Autodesk Fusion 360 part; units mm, degrees
note: some values were not read from the file. Set by a fixed rule: which face or edge a step refers to.
(part 2 of 5)
sketch "Sketch5" plane through (10, 0, 0) normal (1, 0, 0) x (0, 1, 0)
  arc A0 (-151.958, 246.6024) -> (-148.4708, 246.6024) centre (-150.2144, 250.2024) ccw
  line L0 (-151.958, 246.6024) -> (-300.2144, 246.6024)
  line L1 (-300.2144, 246.6024) -> (-300.2144, 240.2024)
  line L2 (-300.2144, 240.2024) -> (249.7856, 240.2024)
  line L3 (249.7856, 240.2024) -> (249.7856, 246.6024)
  line L4 (249.7856, 246.6024) -> (-148.4708, 246.6024)
  line L5 (59.7856, 246.6024) -> (59.7856, 240.2024)
  line L6 (226.7856, 240.2024) -> (226.7856, 243.4024)
  line L7 (235.7856, 240.2024) -> (235.7856, 243.4024)
  line L8 (219.7856, 246.6024) -> (219.7856, 240.2024)
  line L9 (-20.2144, 246.6024) -> (-20.2144, 240.2024)
  line L10 (69.7856, 246.6024) -> (69.7856, 240.2024)
  line L11 (209.7856, 246.6024) -> (209.7856, 240.2024)
  line L12 (-0.2144, 246.6024) -> (-0.2144, 240.2024)
  line L13 (-10.2144, 246.6024) -> (-10.2144, 240.2024)
  line L14 (239.7856, 246.6024) -> (239.7856, 240.2024)
  line L15 (39.7856, 246.6024) -> (39.7856, 240.2024)
  line L16 (232.7856, 240.2024) -> (232.7856, 243.4024)
  line L17 (149.7856, 246.6024) -> (149.7856, 240.2024)
  line L18 (-40.2144, 246.6024) -> (-40.2144, 240.2024)
  line L19 (-50.2144, 246.6024) -> (-50.2144, 240.2024)
  line L20 (29.7856, 246.6024) -> (29.7856, 240.2024)
  line L21 (199.7856, 246.6024) -> (199.7856, 240.2024)
  line L22 (129.7856, 246.6024) -> (129.7856, 240.2024)
  line L23 (224.7856, 240.2024) -> (224.7856, 243.4024)
  line L24 (237.7856, 240.2024) -> (237.7856, 243.4024)
  line L25 (49.7856, 246.6024) -> (49.7856, 240.2024)
  line L26 (218.7856, 240.2024) -> (218.7856, 243.4024)
  line L27 (19.7856, 246.6024) -> (19.7856, 240.2024)
  line L28 (249.7856, 240.2024) -> (249.7856, 246.6024)
  line L29 (159.7856, 246.6024) -> (159.7856, 240.2024)
  line L30 (229.7856, 246.6024) -> (229.7856, 240.2024)
  line L31 (99.7856, 246.6024) -> (99.7856, 240.2024)
  line L32 (249.7856, 246.6024) -> (-120.2144, 246.6024)
  line L33 (169.7856, 246.6024) -> (169.7856, 240.2024)
  line L34 (139.7856, 246.6024) -> (139.7856, 240.2024)
  line L35 (-30.2144, 246.6024) -> (-30.2144, 240.2024)
  line L36 (119.7856, 246.6024) -> (119.7856, 240.2024)
  line L37 (9.7856, 246.6024) -> (9.7856, 240.2024)
  line L38 (-120.2144, 246.6024) -> (-120.2144, 240.2024)
  line L39 (241.7856, 240.2024) -> (241.7856, 243.4024)
  line L40 (231.7856, 240.2024) -> (231.7856, 243.4024)
  line L41 (179.7856, 246.6024) -> (179.7856, 240.2024)
  line L42 (-120.2144, 240.2024) -> (249.7856, 240.2024)
  line L43 (109.7856, 246.6024) -> (109.7856, 240.2024)
  line L44 (189.7856, 246.6024) -> (189.7856, 240.2024)
  line L45 (89.7856, 246.6024) -> (89.7856, 240.2024)
  line L46 (79.7856, 246.6024) -> (79.7856, 240.2024)
  line L47 (205.7856, 240.2024) -> (205.7856, 243.4024)
  line L48 (193.7856, 240.2024) -> (193.7856, 243.4024)
  line L49 (199.7856, 240.2024) -> (199.7856, 243.4024)
  line L50 (238.7856, 240.2024) -> (238.7856, 243.4024)
  line L51 (247.7856, 240.2024) -> (247.7856, 243.4024)
  line L52 (204.7856, 240.2024) -> (204.7856, 243.4024)
  line L53 (223.7856, 240.2024) -> (223.7856, 243.4024)
  line L54 (-90.2144, 246.6024) -> (-90.2144, 240.2024)
  line L55 (215.7856, 240.2024) -> (215.7856, 243.4024)
  line L56 (-70.2144, 246.6024) -> (-70.2144, 240.2024)
  line L57 (246.7856, 240.2024) -> (246.7856, 243.4024)
  line L58 (201.7856, 240.2024) -> (201.7856, 243.4024)
  line L59 (200.7856, 240.2024) -> (200.7856, 243.4024)
  line L60 (245.7856, 240.2024) -> (245.7856, 243.4024)
  line L61 (227.7856, 240.2024) -> (227.7856, 243.4024)
  line L62 (244.7856, 240.2024) -> (244.7856, 243.4024)
  line L63 (140.7856, 240.2024) -> (140.7856, 243.4024)
  line L64 (203.7856, 240.2024) -> (203.7856, 243.4024)
  line L65 (197.7856, 240.2024) -> (197.7856, 243.4024)
  line L66 (211.7856, 240.2024) -> (211.7856, 243.4024)
  line L67 (212.7856, 240.2024) -> (212.7856, 243.4024)
  line L68 (219.7856, 240.2024) -> (219.7856, 243.4024)
  line L69 (198.7856, 240.2024) -> (198.7856, 243.4024)
  line L70 (234.7856, 240.2024) -> (234.7856, 243.4024)
  line L71 (230.7856, 240.2024) -> (230.7856, 243.4024)
  line L72 (202.7856, 240.2024) -> (202.7856, 243.4024)
  line L73 (248.7856, 240.2024) -> (248.7856, 243.4024)
  line L74 (192.7856, 240.2024) -> (192.7856, 243.4024)
  line L75 (249.7856, 240.2024) -> (249.7856, 243.4024)
  line L76 (242.7856, 240.2024) -> (242.7856, 243.4024)
  line L77 (214.7856, 240.2024) -> (214.7856, 243.4024)
  line L78 (243.7856, 240.2024) -> (243.7856, 243.4024)
  line L79 (194.7856, 240.2024) -> (194.7856, 243.4024)
  line L80 (216.7856, 240.2024) -> (216.7856, 243.4024)
  line L81 (-100.2144, 246.6024) -> (-100.2144, 240.2024)
  line L82 (196.7856, 240.2024) -> (196.7856, 243.4024)
  line L83 (208.7856, 240.2024) -> (208.7856, 243.4024)
  line L84 (228.7856, 240.2024) -> (228.7856, 243.4024)
  line L85 (181.7856, 240.2024) -> (181.7856, 243.4024)
  line L86 (171.7856, 240.2024) -> (171.7856, 243.4024)
  line L87 (160.7856, 240.2024) -> (160.7856, 243.4024)
  line L88 (169.7856, 240.2024) -> (169.7856, 243.4024)
  line L89 (151.7856, 240.2024) -> (151.7856, 243.4024)
  line L90 (220.7856, 240.2024) -> (220.7856, 243.4024)
  line L91 (210.7856, 240.2024) -> (210.7856, 243.4024)
  line L92 (185.7856, 240.2024) -> (185.7856, 243.4024)
  line L93 (240.7856, 240.2024) -> (240.7856, 243.4024)
  line L94 (217.7856, 240.2024) -> (217.7856, 243.4024)
  line L95 (233.7856, 240.2024) -> (233.7856, 243.4024)
  line L96 (225.7856, 240.2024) -> (225.7856, 243.4024)
  line L97 (207.7856, 240.2024) -> (207.7856, 243.4024)
  line L98 (158.7856, 240.2024) -> (158.7856, 243.4024)
  line L99 (222.7856, 240.2024) -> (222.7856, 243.4024)
  line L100 (209.7856, 240.2024) -> (209.7856, 243.4024)
  line L101 (-60.2144, 246.6024) -> (-60.2144, 240.2024)
  line L102 (221.7856, 240.2024) -> (221.7856, 243.4024)
  line L103 (-110.2144, 246.6024) -> (-110.2144, 240.2024)
  line L104 (239.7856, 240.2024) -> (239.7856, 243.4024)
  line L105 (-80.2144, 246.6024) -> (-80.2144, 240.2024)
  line L106 (236.7856, 240.2024) -> (236.7856, 243.4024)
  line L107 (229.7856, 240.2024) -> (229.7856, 243.4024)
  line L108 (213.7856, 240.2024) -> (213.7856, 243.4024)
  line L109 (206.7856, 240.2024) -> (206.7856, 243.4024)
  line L110 (195.7856, 240.2024) -> (195.7856, 243.4024)
  line L111 (131.7856, 240.2024) -> (131.7856, 243.4024)
  line L112 (129.7856, 240.2024) -> (129.7856, 243.4024)
  line L113 (177.7856, 240.2024) -> (177.7856, 243.4024)
  line L114 (174.7856, 240.2024) -> (174.7856, 243.4024)
  line L115 (183.7856, 240.2024) -> (183.7856, 243.4024)
  line L116 (179.7856, 240.2024) -> (179.7856, 243.4024)
  line L117 (180.7856, 240.2024) -> (180.7856, 243.4024)
  line L118 (155.7856, 240.2024) -> (155.7856, 243.4024)
  line L119 (191.7856, 240.2024) -> (191.7856, 243.4024)
  line L120 (152.7856, 240.2024) -> (152.7856, 243.4024)
  line L121 (130.7856, 240.2024) -> (130.7856, 243.4024)
  line L122 (190.7856, 240.2024) -> (190.7856, 243.4024)
  line L123 (170.7856, 240.2024) -> (170.7856, 243.4024)
  line L124 (91.7856, 240.2024) -> (91.7856, 243.4024)
  line L125 (122.7856, 240.2024) -> (122.7856, 243.4024)
  line L126 (143.7856, 240.2024) -> (143.7856, 243.4024)
  line L127 (132.7856, 240.2024) -> (132.7856, 243.4024)
  line L128 (184.7856, 240.2024) -> (184.7856, 243.4024)
  line L129 (161.7856, 240.2024) -> (161.7856, 243.4024)
  line L130 (96.7856, 240.2024) -> (96.7856, 243.4024)
  line L131 (84.7856, 240.2024) -> (84.7856, 243.4024)
  line L132 (82.7856, 240.2024) -> (82.7856, 243.4024)
  line L133 (172.7856, 240.2024) -> (172.7856, 243.4024)
  line L134 (92.7856, 240.2024) -> (92.7856, 243.4024)
  line L135 (144.7856, 240.2024) -> (144.7856, 243.4024)
  line L136 (147.7856, 240.2024) -> (147.7856, 243.4024)
  line L137 (81.7856, 240.2024) -> (81.7856, 243.4024)
  line L138 (138.7856, 240.2024) -> (138.7856, 243.4024)
  line L139 (86.7856, 240.2024) -> (86.7856, 243.4024)
  line L140 (149.7856, 240.2024) -> (149.7856, 243.4024)
  line L141 (175.7856, 240.2024) -> (175.7856, 243.4024)
  line L142 (176.7856, 240.2024) -> (176.7856, 243.4024)
  line L143 (182.7856, 240.2024) -> (182.7856, 243.4024)
  line L144 (137.7856, 240.2024) -> (137.7856, 243.4024)
  line L145 (156.7856, 240.2024) -> (156.7856, 243.4024)
  line L146 (128.7856, 240.2024) -> (128.7856, 243.4024)
  line L147 (135.7856, 240.2024) -> (135.7856, 243.4024)
  line L148 (136.7856, 240.2024) -> (136.7856, 243.4024)
  line L149 (167.7856, 240.2024) -> (167.7856, 243.4024)
  line L150 (142.7856, 240.2024) -> (142.7856, 243.4024)
  line L151 (189.7856, 240.2024) -> (189.7856, 243.4024)
  line L152 (133.7856, 240.2024) -> (133.7856, 243.4024)
  line L153 (145.7856, 240.2024) -> (145.7856, 243.4024)
  line L154 (157.7856, 240.2024) -> (157.7856, 243.4024)
  line L155 (173.7856, 240.2024) -> (173.7856, 243.4024)
  line L156 (165.7856, 240.2024) -> (165.7856, 243.4024)
  line L157 (153.7856, 240.2024) -> (153.7856, 243.4024)
  line L158 (159.7856, 240.2024) -> (159.7856, 243.4024)
  line L159 (141.7856, 240.2024) -> (141.7856, 243.4024)
  line L160 (134.7856, 240.2024) -> (134.7856, 243.4024)
  line L161 (166.7856, 240.2024) -> (166.7856, 243.4024)
  line L162 (178.7856, 240.2024) -> (178.7856, 243.4024)
  line L163 (146.7856, 240.2024) -> (146.7856, 243.4024)
  line L164 (186.7856, 240.2024) -> (186.7856, 243.4024)
  line L165 (188.7856, 240.2024) -> (188.7856, 243.4024)
  line L166 (148.7856, 240.2024) -> (148.7856, 243.4024)
  line L167 (154.7856, 240.2024) -> (154.7856, 243.4024)
  line L168 (162.7856, 240.2024) -> (162.7856, 243.4024)
  line L169 (168.7856, 240.2024) -> (168.7856, 243.4024)
  line L170 (164.7856, 240.2024) -> (164.7856, 243.4024)
  line L171 (187.7856, 240.2024) -> (187.7856, 243.4024)
  line L172 (139.7856, 240.2024) -> (139.7856, 243.4024)
  line L173 (150.7856, 240.2024) -> (150.7856, 243.4024)
  line L174 (163.7856, 240.2024) -> (163.7856, 243.4024)
  line L175 (73.7856, 240.2024) -> (73.7856, 243.4024)
  line L176 (71.7856, 240.2024) -> (71.7856, 243.4024)
  line L177 (77.7856, 240.2024) -> (77.7856, 243.4024)
  line L178 (70.7856, 240.2024) -> (70.7856, 243.4024)
  line L179 (88.7856, 240.2024) -> (88.7856, 243.4024)
  line L180 (85.7856, 240.2024) -> (85.7856, 243.4024)
  line L181 (67.7856, 240.2024) -> (67.7856, 243.4024)
  line L182 (99.7856, 240.2024) -> (99.7856, 243.4024)
  line L183 (98.7856, 240.2024) -> (98.7856, 243.4024)
  line L184 (68.7856, 240.2024) -> (68.7856, 243.4024)
  line L185 (87.7856, 240.2024) -> (87.7856, 243.4024)
  line L186 (120.7856, 240.2024) -> (120.7856, 243.4024)
  line L187 (112.7856, 240.2024) -> (112.7856, 243.4024)
  line L188 (101.7856, 240.2024) -> (101.7856, 243.4024)
  line L189 (104.7856, 240.2024) -> (104.7856, 243.4024)
  line L190 (64.7856, 240.2024) -> (64.7856, 243.4024)
  line L191 (72.7856, 240.2024) -> (72.7856, 243.4024)
  line L192 (78.7856, 240.2024) -> (78.7856, 243.4024)
  line L193 (127.7856, 240.2024) -> (127.7856, 243.4024)
  line L194 (49.7856, 240.2024) -> (49.7856, 243.4024)
  line L195 (36.7856, 240.2024) -> (36.7856, 243.4024)
  line L196 (62.7856, 240.2024) -> (62.7856, 243.4024)
  line L197 (119.7856, 240.2024) -> (119.7856, 243.4024)
  line L198 (39.7856, 240.2024) -> (39.7856, 243.4024)
  line L199 (65.7856, 240.2024) -> (65.7856, 243.4024)
  line L200 (56.7856, 240.2024) -> (56.7856, 243.4024)
  line L201 (28.7856, 240.2024) -> (28.7856, 243.4024)
  line L202 (51.7856, 240.2024) -> (51.7856, 243.4024)
  line L203 (54.7856, 240.2024) -> (54.7856, 243.4024)
  line L204 (126.7856, 240.2024) -> (126.7856, 243.4024)
  line L205 (116.7856, 240.2024) -> (116.7856, 243.4024)
  line L206 (110.7856, 240.2024) -> (110.7856, 243.4024)
  line L207 (102.7856, 240.2024) -> (102.7856, 243.4024)
  line L208 (95.7856, 240.2024) -> (95.7856, 243.4024)
  line L209 (79.7856, 240.2024) -> (79.7856, 243.4024)
  line L210 (117.7856, 240.2024) -> (117.7856, 243.4024)
  line L211 (69.7856, 240.2024) -> (69.7856, 243.4024)
  line L212 (124.7856, 240.2024) -> (124.7856, 243.4024)
  line L213 (80.7856, 240.2024) -> (80.7856, 243.4024)
  line L214 (123.7856, 240.2024) -> (123.7856, 243.4024)
  line L215 (107.7856, 240.2024) -> (107.7856, 243.4024)
  line L216 (66.7856, 240.2024) -> (66.7856, 243.4024)
  line L217 (113.7856, 240.2024) -> (113.7856, 243.4024)
  line L218 (76.7856, 240.2024) -> (76.7856, 243.4024)
  line L219 (89.7856, 240.2024) -> (89.7856, 243.4024)
  line L220 (105.7856, 240.2024) -> (105.7856, 243.4024)
  line L221 (121.7856, 240.2024) -> (121.7856, 243.4024)
  line L222 (106.7856, 240.2024) -> (106.7856, 243.4024)
  line L223 (118.7856, 240.2024) -> (118.7856, 243.4024)
  line L224 (109.7856, 240.2024) -> (109.7856, 243.4024)
  line L225 (115.7856, 240.2024) -> (115.7856, 243.4024)
  line L226 (114.7856, 240.2024) -> (114.7856, 243.4024)
  line L227 (94.7856, 240.2024) -> (94.7856, 243.4024)
  line L228 (74.7856, 240.2024) -> (74.7856, 243.4024)
  line L229 (93.7856, 240.2024) -> (93.7856, 243.4024)
  line L230 (111.7856, 240.2024) -> (111.7856, 243.4024)
  line L231 (75.7856, 240.2024) -> (75.7856, 243.4024)
  line L232 (103.7856, 240.2024) -> (103.7856, 243.4024)
  line L233 (83.7856, 240.2024) -> (83.7856, 243.4024)
  line L234 (125.7856, 240.2024) -> (125.7856, 243.4024)
  line L235 (97.7856, 240.2024) -> (97.7856, 243.4024)
  line L236 (100.7856, 240.2024) -> (100.7856, 243.4024)
  line L237 (90.7856, 240.2024) -> (90.7856, 243.4024)
  line L238 (108.7856, 240.2024) -> (108.7856, 243.4024)
  line L239 (24.7856, 240.2024) -> (24.7856, 243.4024)
  line L240 (19.7856, 240.2024) -> (19.7856, 243.4024)
  line L241 (61.7856, 240.2024) -> (61.7856, 243.4024)
  line L242 (17.7856, 240.2024) -> (17.7856, 243.4024)
  line L243 (26.7856, 240.2024) -> (26.7856, 243.4024)
  line L244 (45.7856, 240.2024) -> (45.7856, 243.4024)
  line L245 (38.7856, 240.2024) -> (38.7856, 243.4024)
  line L246 (14.7856, 240.2024) -> (14.7856, 243.4024)
  line L247 (32.7856, 240.2024) -> (32.7856, 243.4024)
  line L248 (23.7856, 240.2024) -> (23.7856, 243.4024)
  line L249 (44.7856, 240.2024) -> (44.7856, 243.4024)
  line L250 (27.7856, 240.2024) -> (27.7856, 243.4024)
  line L251 (60.7856, 240.2024) -> (60.7856, 243.4024)
  line L252 (50.7856, 240.2024) -> (50.7856, 243.4024)
  line L253 (58.7856, 240.2024) -> (58.7856, 243.4024)
  line L254 (8.7856, 240.2024) -> (8.7856, 243.4024)
  line L255 (57.7856, 240.2024) -> (57.7856, 243.4024)
  line L256 (-38.2144, 240.2024) -> (-38.2144, 243.4024)
  line L257 (7.7856, 240.2024) -> (7.7856, 243.4024)
  line L258 (47.7856, 240.2024) -> (47.7856, 243.4024)
  line L259 (10.7856, 240.2024) -> (10.7856, 243.4024)
  line L260 (35.7856, 240.2024) -> (35.7856, 243.4024)
  line L261 (25.7856, 240.2024) -> (25.7856, 243.4024)
  line L262 (43.7856, 240.2024) -> (43.7856, 243.4024)
  line L263 (2.7856, 240.2024) -> (2.7856, 243.4024)
  line L264 (1.7856, 240.2024) -> (1.7856, 243.4024)
  line L265 (5.7856, 240.2024) -> (5.7856, 243.4024)
  line L266 (42.7856, 240.2024) -> (42.7856, 243.4024)
  line L267 (18.7856, 240.2024) -> (18.7856, 243.4024)
  line L268 (53.7856, 240.2024) -> (53.7856, 243.4024)
  line L269 (46.7856, 240.2024) -> (46.7856, 243.4024)
  line L270 (52.7856, 240.2024) -> (52.7856, 243.4024)
  line L271 (59.7856, 240.2024) -> (59.7856, 243.4024)
  line L272 (0.7856, 240.2024) -> (0.7856, 243.4024)
  line L273 (6.7856, 240.2024) -> (6.7856, 243.4024)
  line L274 (22.7856, 240.2024) -> (22.7856, 243.4024)
  line L275 (21.7856, 240.2024) -> (21.7856, 243.4024)
  line L276 (29.7856, 240.2024) -> (29.7856, 243.4024)
  line L277 (37.7856, 240.2024) -> (37.7856, 243.4024)
  line L278 (55.7856, 240.2024) -> (55.7856, 243.4024)
  line L279 (3.7856, 240.2024) -> (3.7856, 243.4024)
  line L280 (41.7856, 240.2024) -> (41.7856, 243.4024)
  line L281 (4.7856, 240.2024) -> (4.7856, 243.4024)
  line L282 (11.7856, 240.2024) -> (11.7856, 243.4024)
  line L283 (-3.2144, 240.2024) -> (-3.2144, 243.4024)
  line L284 (-40.2144, 240.2024) -> (-40.2144, 243.4024)
  line L285 (16.7856, 240.2024) -> (16.7856, 243.4024)
  line L286 (13.7856, 240.2024) -> (13.7856, 243.4024)
  line L287 (30.7856, 240.2024) -> (30.7856, 243.4024)
  line L288 (-35.2144, 240.2024) -> (-35.2144, 243.4024)
  line L289 (-44.2144, 240.2024) -> (-44.2144, 243.4024)
  line L290 (-49.2144, 240.2024) -> (-49.2144, 243.4024)
  line L291 (9.7856, 240.2024) -> (9.7856, 243.4024)
  line L292 (-9.2144, 240.2024) -> (-9.2144, 243.4024)
  line L293 (12.7856, 240.2024) -> (12.7856, 243.4024)
  line L294 (48.7856, 240.2024) -> (48.7856, 243.4024)
  line L295 (20.7856, 240.2024) -> (20.7856, 243.4024)
  line L296 (63.7856, 240.2024) -> (63.7856, 243.4024)
  line L297 (-27.2144, 240.2024) -> (-27.2144, 243.4024)
  line L298 (15.7856, 240.2024) -> (15.7856, 243.4024)
  line L299 (40.7856, 240.2024) -> (40.7856, 243.4024)
  line L300 (31.7856, 240.2024) -> (31.7856, 243.4024)
  line L301 (33.7856, 240.2024) -> (33.7856, 243.4024)
  line L302 (34.7856, 240.2024) -> (34.7856, 243.4024)
  line L303 (-26.2144, 240.2024) -> (-26.2144, 243.4024)
  line L304 (-48.2144, 240.2024) -> (-48.2144, 243.4024)
  line L305 (-110.2144, 240.2024) -> (-110.2144, 243.4024)
  line L306 (-53.2144, 240.2024) -> (-53.2144, 243.4024)
  line L307 (-10.2144, 240.2024) -> (-10.2144, 243.4024)
  line L308 (-13.2144, 240.2024) -> (-13.2144, 243.4024)
  line L309 (-21.2144, 240.2024) -> (-21.2144, 243.4024)
  line L310 (-58.2144, 240.2024) -> (-58.2144, 243.4024)
  line L311 (-60.2144, 240.2024) -> (-60.2144, 243.4024)
  line L312 (-63.2144, 240.2024) -> (-63.2144, 243.4024)
  line L313 (-45.2144, 240.2024) -> (-45.2144, 243.4024)
  line L314 (-5.2144, 240.2024) -> (-5.2144, 243.4024)
  line L315 (-11.2144, 240.2024) -> (-11.2144, 243.4024)
  line L316 (-54.2144, 240.2024) -> (-54.2144, 243.4024)
  line L317 (-24.2144, 240.2024) -> (-24.2144, 243.4024)
  line L318 (-43.2144, 240.2024) -> (-43.2144, 243.4024)
  line L319 (-59.2144, 240.2024) -> (-59.2144, 243.4024)
  line L320 (-46.2144, 240.2024) -> (-46.2144, 243.4024)
  line L321 (-36.2144, 240.2024) -> (-36.2144, 243.4024)
  line L322 (-22.2144, 240.2024) -> (-22.2144, 243.4024)
  line L323 (-16.2144, 240.2024) -> (-16.2144, 243.4024)
  line L324 (-30.2144, 240.2024) -> (-30.2144, 243.4024)
  line L325 (-57.2144, 240.2024) -> (-57.2144, 243.4024)
  line L326 (-0.2144, 240.2024) -> (-0.2144, 243.4024)
  line L327 (-19.2144, 240.2024) -> (-19.2144, 243.4024)
  line L328 (-51.2144, 240.2024) -> (-51.2144, 243.4024)
  line L329 (-1.2144, 240.2024) -> (-1.2144, 243.4024)
  line L330 (-6.2144, 240.2024) -> (-6.2144, 243.4024)
  line L331 (-47.2144, 240.2024) -> (-47.2144, 243.4024)
  line L332 (-33.2144, 240.2024) -> (-33.2144, 243.4024)
  line L333 (-17.2144, 240.2024) -> (-17.2144, 243.4024)
  line L334 (-37.2144, 240.2024) -> (-37.2144, 243.4024)
  line L335 (-52.2144, 240.2024) -> (-52.2144, 243.4024)
  line L336 (-18.2144, 240.2024) -> (-18.2144, 243.4024)
  line L337 (-23.2144, 240.2024) -> (-23.2144, 243.4024)
  line L338 (-82.2144, 240.2024) -> (-82.2144, 243.4024)
  line L339 (-95.2144, 240.2024) -> (-95.2144, 243.4024)
  line L340 (-71.2144, 240.2024) -> (-71.2144, 243.4024)
  line L341 (-14.2144, 240.2024) -> (-14.2144, 243.4024)
  line L342 (-7.2144, 240.2024) -> (-7.2144, 243.4024)
  line L343 (-56.2144, 240.2024) -> (-56.2144, 243.4024)
  line L344 (-39.2144, 240.2024) -> (-39.2144, 243.4024)
  line L345 (-25.2144, 240.2024) -> (-25.2144, 243.4024)
  line L346 (-4.2144, 240.2024) -> (-4.2144, 243.4024)
  line L347 (-55.2144, 240.2024) -> (-55.2144, 243.4024)
  line L348 (-32.2144, 240.2024) -> (-32.2144, 243.4024)
  line L349 (-8.2144, 240.2024) -> (-8.2144, 243.4024)
  line L350 (-29.2144, 240.2024) -> (-29.2144, 243.4024)
  line L351 (-42.2144, 240.2024) -> (-42.2144, 243.4024)
  line L352 (-34.2144, 240.2024) -> (-34.2144, 243.4024)
  line L353 (-2.2144, 240.2024) -> (-2.2144, 243.4024)
  line L354 (-62.2144, 240.2024) -> (-62.2144, 243.4024)
  line L355 (-61.2144, 240.2024) -> (-61.2144, 243.4024)
  line L356 (-15.2144, 240.2024) -> (-15.2144, 243.4024)
  line L357 (-28.2144, 240.2024) -> (-28.2144, 243.4024)
  line L358 (-50.2144, 240.2024) -> (-50.2144, 243.4024)
  line L359 (-31.2144, 240.2024) -> (-31.2144, 243.4024)
  line L360 (-64.2144, 240.2024) -> (-64.2144, 243.4024)
  line L361 (-74.2144, 240.2024) -> (-74.2144, 243.4024)
  line L362 (-12.2144, 240.2024) -> (-12.2144, 243.4024)
  line L363 (-20.2144, 240.2024) -> (-20.2144, 243.4024)
  line L364 (-41.2144, 240.2024) -> (-41.2144, 243.4024)
  line L365 (-108.2144, 240.2024) -> (-108.2144, 243.4024)
  line L366 (-75.2144, 240.2024) -> (-75.2144, 243.4024)
  line L367 (-83.2144, 240.2024) -> (-83.2144, 243.4024)
  line L368 (-80.2144, 240.2024) -> (-80.2144, 243.4024)
  line L369 (-117.2144, 240.2024) -> (-117.2144, 243.4024)
  line L370 (-86.2144, 240.2024) -> (-86.2144, 243.4024)
  line L371 (-100.2144, 240.2024) -> (-100.2144, 243.4024)
  line L372 (-72.2144, 240.2024) -> (-72.2144, 243.4024)
  line L373 (-114.2144, 240.2024) -> (-114.2144, 243.4024)
  line L374 (-91.2144, 240.2024) -> (-91.2144, 243.4024)
  line L375 (-88.2144, 240.2024) -> (-88.2144, 243.4024)
  line L376 (-79.2144, 240.2024) -> (-79.2144, 243.4024)
  line L377 (-112.2144, 240.2024) -> (-112.2144, 243.4024)
  line L378 (-104.2144, 240.2024) -> (-104.2144, 243.4024)
  line L379 (-96.2144, 240.2024) -> (-96.2144, 243.4024)
  line L380 (-111.2144, 240.2024) -> (-111.2144, 243.4024)
  line L381 (-69.2144, 240.2024) -> (-69.2144, 243.4024)
  line L382 (-76.2144, 240.2024) -> (-76.2144, 243.4024)
  line L383 (-70.2144, 240.2024) -> (-70.2144, 243.4024)
  line L384 (-115.2144, 240.2024) -> (-115.2144, 243.4024)
  line L385 (-89.2144, 240.2024) -> (-89.2144, 243.4024)
  line L386 (-92.2144, 240.2024) -> (-92.2144, 243.4024)
  line L387 (-84.2144, 240.2024) -> (-84.2144, 243.4024)
  line L388 (-98.2144, 240.2024) -> (-98.2144, 243.4024)
  line L389 (-94.2144, 240.2024) -> (-94.2144, 243.4024)
  line L390 (-113.2144, 240.2024) -> (-113.2144, 243.4024)
  line L391 (-93.2144, 240.2024) -> (-93.2144, 243.4024)
  line L392 (-99.2144, 240.2024) -> (-99.2144, 243.4024)
  line L393 (-87.2144, 240.2024) -> (-87.2144, 243.4024)
  line L394 (-97.2144, 240.2024) -> (-97.2144, 243.4024)
  line L395 (-116.2144, 240.2024) -> (-116.2144, 243.4024)
  line L396 (-90.2144, 240.2024) -> (-90.2144, 243.4024)
  line L397 (-109.2144, 240.2024) -> (-109.2144, 243.4024)
  line L398 (-102.2144, 240.2024) -> (-102.2144, 243.4024)
  line L399 (-105.2144, 240.2024) -> (-105.2144, 243.4024)
  line L400 (-106.2144, 240.2024) -> (-106.2144, 243.4024)
  line L401 (-103.2144, 240.2024) -> (-103.2144, 243.4024)
  line L402 (-68.2144, 240.2024) -> (-68.2144, 243.4024)
  line L403 (-66.2144, 240.2024) -> (-66.2144, 243.4024)
  line L404 (-85.2144, 240.2024) -> (-85.2144, 243.4024)
  line L405 (-65.2144, 240.2024) -> (-65.2144, 243.4024)
  line L406 (-107.2144, 240.2024) -> (-107.2144, 243.4024)
  line L407 (-101.2144, 240.2024) -> (-101.2144, 243.4024)
  line L408 (-67.2144, 240.2024) -> (-67.2144, 243.4024)
  line L409 (-78.2144, 240.2024) -> (-78.2144, 243.4024)
  line L410 (-77.2144, 240.2024) -> (-77.2144, 243.4024)
  line L411 (-81.2144, 240.2024) -> (-81.2144, 243.4024)
  line L412 (-73.2144, 240.2024) -> (-73.2144, 243.4024)
  line L413 (-119.2144, 240.2024) -> (-119.2144, 243.4024)
  line L414 (-118.2144, 240.2024) -> (-118.2144, 243.4024)
component "Component" placed x (1, 0, 0) y (0, 0, -1) z (0, 1, 0) at (0, -250.2144, 250.2024)
equation "length = 500 mm"
equation "d57 = length"
equation "holeLocation = 100 mm"
equation "d60 = holeLocation"

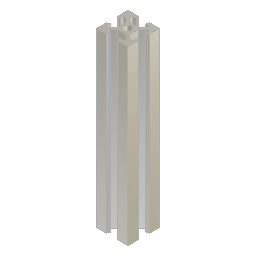
design "stop"
Autodesk Fusion 360 part; units mm, degrees
sketch "Sketch1" plane through (0, 0, 0) normal (0, 0, 1) x (1, 0, 0)
  line L0 (-10, 10) -> (10, 10) construction
  line L1 (10, 10) -> (10, -10) construction
  line L2 (10, -10) -> (-10, -10) construction
  line L3 (-10, -10) -> (-10, 10) construction
  circle A0 centre (0, 0) radius 2.5
  line L4 (0, -10) -> (0, -3.9) construction
  line L5 (-10, 0) -> (-3.9, 0) construction
  line L6 (10, 0) -> (3.9, 0) construction
  line L7 (0, 10) -> (0, 3.9) construction
  line L8 (3.9, 3.6) -> (3.9, 0) construction
  line L9 (3.9, -3.0515) -> (3.9, 3.1)
  line L10 (-3.9, 3.1) -> (-3.9, -3.0515)
  line L11 (10, 10) -> (-10, -10) construction
  line L12 (-10, 10) -> (10, -10) construction
  line L13 (3.9, 3.9) -> (4.3243, 3.4757) construction
  line L14 (3.9, 3.9) -> (3.4757, 4.3243) construction
  line L15 (-3.9, 3.9) -> (-3.4757, 4.3243) construction
  line L16 (-3.4757, 4.3243) -> (-4.3243, 3.4757) construction
  line L17 (-3.9, -3.9) -> (-4.3243, -3.4757) construction
  line L18 (-4.3243, -3.4757) -> (-3.4757, -4.3243) construction
  line L19 (3.9, -3.9) -> (4.3243, -3.4757) construction
  line L20 (4.3243, -3.4757) -> (3.4757, -4.3243) construction
  line L21 (3.4757, -4.3243) -> (3.0515, -3.9)
  line L22 (4.3243, -3.4757) -> (3.9, -3.0515)
  line L23 (10, -10) -> (9.1515, -10)
  line L24 (10, -9.1515) -> (10, -10)
  line L25 (3.4757, 4.3243) -> (3.0515, 3.9)
  line L26 (3.4757, 4.3243) -> (2.8757, 4.3243) construction
  line L27 (4.3243, 3.4757) -> (3.9, 3.0515)
  line L28 (-4.3243, 3.4757) -> (-3.9, 3.0515)
  line L29 (-3.4757, 4.3243) -> (-3.0515, 3.9)
  line L30 (-3.4757, -4.3243) -> (-3.0515, -3.9)
  line L31 (-4.3243, -3.4757) -> (-3.9, -3.0515)
  line L32 (-4.3243, -3.4757) -> (-3.7243, -3.4757) construction
  line L33 (-9.1515, -10) -> (-10, -10)
  line L34 (-10, -10) -> (-10, -9.1515)
  line L35 (-10, 9.1515) -> (-10, 10)
  line L36 (-10, 10) -> (-9.1515, 10)
  line L37 (9.1515, 10) -> (10, 10)
  line L38 (10, 9.1515) -> (10, 10)
  line L39 (10, -10) -> (8.2, -10) construction
  line L40 (8.2, -10) -> (8.2, -8.2) construction
  line L41 (8.2, -8.2) -> (10, -8.2) construction
  line L42 (10, -8.2) -> (10, -10) construction
  line L43 (-10, -10) -> (-8.2, -10) construction
  line L44 (-8.2, -10) -> (-8.2, -8.2) construction
  line L45 (-8.2, -8.2) -> (-10, -8.2) construction
  line L46 (-10, -8.2) -> (-10, -10) construction
  line L47 (-10, 10) -> (-8.2, 10) construction
  line L48 (-8.2, 10) -> (-8.2, 8.2) construction
  line L49 (-8.2, 8.2) -> (-10, 8.2) construction
  line L50 (-10, 8.2) -> (-10, 10) construction
  line L51 (10, 10) -> (8.2, 10) construction
  line L52 (8.2, 10) -> (8.2, 8.2) construction
  line L53 (8.2, 8.2) -> (10, 8.2) construction
  line L54 (10, 8.2) -> (10, 10) construction
  line L55 (-10, -10) -> (-9.1, -10) construction
  line L56 (-9.1, -10) -> (-9.1, -9.1) construction
  line L57 (-9.1, -9.1) -> (-10, -9.1) construction
  line L58 (-10, -9.1) -> (-10, -10) construction
  line L59 (-10, 10) -> (-9.1, 10) construction
  line L60 (-9.1, 10) -> (-9.1, 9.1) construction
  line L61 (-9.1, 9.1) -> (-10, 9.1) construction
  line L62 (-10, 9.1) -> (-10, 10) construction
  line L63 (10, 10) -> (9.1, 10) construction
  line L64 (9.1, 10) -> (9.1, 9.1) construction
  line L65 (9.1, 9.1) -> (10, 9.1) construction
  line L66 (10, 9.1) -> (10, 10) construction
  line L67 (10, -10) -> (9.1, -10) construction
  line L68 (9.1, -10) -> (9.1, -9.1) construction
  line L69 (9.1, -9.1) -> (10, -9.1) construction
  line L70 (10, -9.1) -> (10, -10) construction
  line L71 (0, -10) -> (3.1, -10) construction
  line L72 (3.1, -10) -> (-3, -10) construction
  line L73 (-3, -10) -> (-3, 10) construction
  line L74 (-3, 10) -> (3.1, 10) construction
  line L75 (3.1, 10) -> (3.1, -10) construction
  line L76 (-10, 0) -> (-10, 3.1) construction
  line L77 (-10, 3.1) -> (10, 3.1) construction
  line L78 (10, 3.1) -> (10, -3) construction
  line L79 (10, -3) -> (-10, -3) construction
  line L80 (-10, -3) -> (-10, 3.1) construction
  line L81 (0, -10) -> (-5.45, -10) construction
  line L82 (-5.45, -10) -> (5.45, -10) construction
  line L83 (5.45, 10) -> (-5.45, 10) construction
  line L84 (-10, 0) -> (-10, 5.45) construction
  line L85 (10, 5.45) -> (10, -5.45) construction
  line L86 (-10, -5.45) -> (-10, 5.45) construction
  line L87 (-10, -10) -> (-5.45, -10)
  line L88 (-10, -5.45) -> (-10, -10)
  line L89 (10, -10) -> (5.45, -10)
  line L90 (10, -5.45) -> (10, -10)
  line L91 (10, 10) -> (5.45, 10)
  line L92 (5.45, 8.2) -> (5.45, 6.2985)
  line L93 (10, 5.45) -> (10, 10)
  line L94 (-10, 10) -> (-5.45, 10)
  line L95 (-5.45, 8.2) -> (-5.45, 6.2985)
  line L96 (-6.2985, 5.45) -> (-8.2, 5.45)
  line L97 (-10, 5.45) -> (-10, 10)
  line L98 (10, 0) -> (10, 3.6) construction
  line L99 (-10, 3.6) -> (-10, -3.6) construction
  line L100 (10, -3.6) -> (10, 3.6) construction
  line L101 (0, 10) -> (-3.6, 10) construction
  line L102 (-3.6, 10) -> (3.6, 10) construction
  line L103 (3.6, -10) -> (-3.6, -10) construction
  line L104 (-8.2, -8.2) -> (8.2, -8.2) construction
  line L105 (8.2, -8.2) -> (8.2, 8.2) construction
  line L106 (8.2, 8.2) -> (-8.2, 8.2) construction
  line L107 (-8.2, 8.2) -> (-8.2, -8.2) construction
  line L108 (-5.45, -10) -> (-3.6, -10)
  line L109 (-3.6, -10) -> (-3.6, -9.1)
  line L110 (-3.6, -8.2) -> (-5.45, -8.2)
  line L111 (-10, -3.6) -> (-9.1, -3.6)
  line L112 (-8.2, -3.6) -> (-8.2, -5.45)
  line L113 (-10, -5.45) -> (-10, -3.6)
  line L114 (-9.1, 3.6) -> (-10, 3.6)
  line L115 (-10, 3.6) -> (-10, 5.45)
  line L116 (-8.2, 5.45) -> (-8.2, 3.6)
  line L117 (3.6, 8.2) -> (5.45, 8.2)
  line L118 (5.45, 10) -> (3.6, 10)
  line L119 (3.6, 10) -> (3.6, 9.1)
  line L120 (-5.45, 10) -> (-3.6, 10)
  line L121 (-3.6, 10) -> (-3.6, 9.1)
  line L122 (-3.6, 8.2) -> (-5.45, 8.2)
  line L123 (10, 5.45) -> (10, 3.6)
  line L124 (10, 3.6) -> (9.1, 3.6)
  line L125 (8.2, 3.6) -> (8.2, 5.45)
  line L126 (10, -5.45) -> (10, -3.6)
  line L127 (10, -3.6) -> (9.1, -3.6)
  line L128 (8.2, -3.6) -> (8.2, -5.45)
  line L129 (5.45, -8.2) -> (3.6, -8.2)
  line L130 (3.6, -9.1) -> (3.6, -10)
  line L131 (3.6, -10) -> (5.45, -10)
  line L132 (9.1, -9.1) -> (-9.1, -9.1) construction
  line L133 (-9.1, -9.1) -> (-9.1, 9.1) construction
  line L134 (-9.1, 9.1) -> (9.1, 9.1) construction
  line L135 (9.1, 9.1) -> (9.1, -9.1) construction
  line L136 (3.6, -9.1) -> (3.1, -9.1)
  line L137 (3.1, -9.1) -> (3.1, -8.2)
  line L138 (3.1, -8.2) -> (3.6, -8.2)
  line L139 (-3, -9.1) -> (-3.6, -9.1)
  line L140 (-3.6, -8.2) -> (-3, -8.2)
  line L141 (-3, -8.2) -> (-3, -9.1)
  line L142 (-8.2, -3.6) -> (-8.2, -3)
  line L143 (-8.2, -3) -> (-9.1, -3)
  line L144 (-9.1, -3) -> (-9.1, -3.6)
  line L145 (-8.2, 3.6) -> (-8.2, 3.1)
  line L146 (-8.2, 3.1) -> (-9.1, 3.1)
  line L147 (-9.1, 3.1) -> (-9.1, 3.6)
  line L148 (-3.6, 9.1) -> (-3, 9.1)
  line L149 (-3, 9.1) -> (-3, 8.2)
  line L150 (-3, 8.2) -> (-3.6, 8.2)
  line L151 (3.1, 9.1) -> (3.6, 9.1)
  line L152 (3.6, 8.2) -> (3.1, 8.2)
  line L153 (3.1, 8.2) -> (3.1, 9.1)
  line L154 (9.1, 3.6) -> (9.1, 3.1)
  line L155 (9.1, 3.1) -> (8.2, 3.1)
  line L156 (8.2, 3.1) -> (8.2, 3.6)
  line L157 (9.1, -3.6) -> (9.1, -3)
  line L158 (9.1, -3) -> (8.2, -3)
  line L159 (8.2, -3) -> (8.2, -3.6)
  line L160 (-3.4757, 4.3243) -> (-5.45, 6.2985)
  line L161 (-4.3243, 3.4757) -> (-6.2985, 5.45)
  line L162 (-3.6, 9.1) -> (-3.6, 10) construction
  line L163 (-9.1, 3.6) -> (-10, 3.6) construction
  line L164 (-3.0515, -3.9) -> (3.1, -3.9)
  line L165 (-3.9, 0) -> (-3.9, -3.0515) construction
  line L166 (0, 3.9) -> (3.1, 3.9) construction
  line L167 (3.1, 3.9) -> (-3.0515, 3.9)
  line L168 (-4.3243, -3.4757) -> (-6.2985, -5.45)
  line L169 (-3.4757, -4.3243) -> (-5.45, -6.2985)
  line L170 (-6.2985, -5.45) -> (-8.2, -5.45)
  line L171 (-10, -3.6) -> (-9.1, -3.6) construction
  line L172 (-5.45, -8.2) -> (-5.45, -6.2985)
  line L173 (-3.6, -10) -> (-3.6, -9.1) construction
  line L174 (-3.6, -8.2) -> (-3.6, 8.2) construction
  line L175 (6.2985, -5.45) -> (8.2, -5.45)
  line L176 (-8.2, -3.6) -> (8.2, -3.6) construction
  line L177 (9.1, -3.6) -> (10, -3.6) construction
  line L178 (3.4757, -4.3243) -> (5.45, -6.2985)
  line L179 (8.2, -9.0485) -> (8.2515, -9.1)
  line L180 (9.1, -9.9485) -> (9.1515, -10)
  line L181 (9.9485, -9.1) -> (10, -9.1515)
  line L182 (4.3243, -3.4757) -> (6.2985, -5.45)
  line L183 (9.0485, -8.2) -> (9.1, -8.2515)
  line L184 (5.45, -8.2) -> (5.45, -6.2985)
  line L185 (6.2985, 5.45) -> (8.2, 5.45)
  line L186 (10, 3.6) -> (9.1, 3.6) construction
  line L187 (8.2, 3.6) -> (-8.2, 3.6) construction
  line L188 (3.4757, 4.3243) -> (5.45, 6.2985)
  line L189 (4.3243, 3.4757) -> (6.2985, 5.45)
  line L190 (3.6, 10) -> (3.6, 9.1) construction
  line L191 (3.6, 8.2) -> (3.6, -10) construction
  dimension "d1" = 20
  dimension "d2" = 20
  dimension "d3" = 5
  dimension "d4" = 6.1
  dimension "d5" = 6.1
  dimension "d6" = 6.1
  dimension "d7" = 6.1
  dimension "d8" = 0.6
  dimension "d9" = 0.6
  dimension "d10" = 0.6
  dimension "d11" = 1.2
  dimension "d12" = 0.6
  dimension "d13" = 1.2
  dimension "d14" = 0.6
  dimension "d15" = 1.2
  dimension "d18" = 45
  dimension "d20" = 45
  dimension "d24" = 1.8
  dimension "d25" = 1.8
  dimension "d26" = 1.8
  dimension "d27" = 1.8
  dimension "d28" = 1.8
  dimension "d29" = 1.8
  dimension "d30" = 1.8
  dimension "d31" = 1.8
  dimension "d32" = 0.9
  dimension "d33" = 0.9
  dimension "d34" = 0.9
  dimension "d35" = 0.9
  dimension "d36" = 0.9
  dimension "d37" = 0.9
  dimension "d38" = 0.9
  dimension "d39" = 0.9
  dimension "d40" = 3.1
  dimension "d41" = 6.1
  dimension "d42" = 3.1
  dimension "d43" = 20
  dimension "d44" = 6.1
  dimension "d47" = 5.45
  dimension "d48" = 10.9
  dimension "d49" = 3.6
  dimension "d50" = 7.2
  dimension "d51" = 20
  dimension "d52" = 3.6
  dimension "d53" = 7.2
  dimension "d54" = 20
  constraint horizontal L0
  constraint vertical L1
  constraint horizontal L2
  constraint vertical L3
  constraint coincident A0.centre origin
  constraint midpoint L2 L4.start
  constraint perpendicular L2 L4
  constraint midpoint L3 L5.start
  constraint perpendicular L3 L5
  constraint perpendicular L5 L165
  constraint midpoint L1 L6.start
  constraint perpendicular L1 L6
  constraint midpoint L0 L7.start
  constraint perpendicular L0 L7
  constraint perpendicular L7 L166
  constraint perpendicular L6 L8
  constraint vertical L9
  constraint vertical L10
  constraint parallel L12 L13
  constraint perpendicular L11 L14
  constraint perpendicular L12 L15
  constraint perpendicular L12 L16
  constraint perpendicular L11 L17
  constraint perpendicular L11 L18
  constraint perpendicular L12 L19
  constraint perpendicular L12 L20
  constraint coincident L2 L23.end
  constraint perpendicular L20 L178
  constraint perpendicular L20 L21
  constraint perpendicular L19 L22
  constraint coincident L1 L24.start
  constraint perpendicular L19 L182
  constraint perpendicular L1 L23
  constraint perpendicular L2 L24
  constraint coincident L1 L38.start
  constraint coincident L0 L37.start
  constraint horizontal L26
  constraint coincident L25.end L166
  constraint coincident L8 L27.end
  constraint coincident L10 L28.end
  constraint perpendicular L16 L28
  constraint perpendicular L16 L29
  constraint perpendicular L18 L30
  constraint horizontal L32
  constraint coincident L3 L34.end
  constraint perpendicular L17 L168
  constraint coincident L2 L33.start
  constraint perpendicular L33 L34
  constraint coincident L3 L35.start
  constraint coincident L0 L36.end
  constraint horizontal L39
  constraint vertical L40
  constraint horizontal L41
  constraint vertical L42
  constraint horizontal L43
  constraint vertical L44
  constraint horizontal L45
  constraint vertical L46
  constraint horizontal L47
  constraint vertical L48
  constraint horizontal L49
  constraint vertical L50
  constraint horizontal L51
  constraint vertical L52
  constraint horizontal L53
  constraint vertical L54
  constraint horizontal L55
  constraint vertical L56
  constraint horizontal L57
  constraint vertical L58
  constraint horizontal L59
  constraint vertical L60
  constraint horizontal L61
  constraint vertical L62
  constraint horizontal L63
  constraint vertical L64
  constraint horizontal L65
  constraint vertical L66
  constraint horizontal L67
  constraint vertical L68
  constraint horizontal L69
  constraint vertical L70
  constraint coincident L2 L71.end
  constraint horizontal L72
  constraint vertical L73
  constraint horizontal L74
  constraint vertical L75
  constraint coincident L0 L73.end
  constraint perpendicular L5 L76
  constraint horizontal L77
  constraint vertical L78
  constraint horizontal L79
  constraint vertical L80
  constraint coincident L2 L81.end
  constraint horizontal L82
  constraint horizontal L83
  constraint coincident L0 L83.start
  constraint perpendicular L5 L84
  constraint vertical L85
  constraint vertical L86
  constraint coincident L1 L85.end
  constraint horizontal L87
  constraint horizontal L170
  constraint vertical L88
  constraint horizontal L89
  constraint horizontal L175
  constraint vertical L90
  constraint horizontal L91
  constraint vertical L92
  constraint horizontal L185
  constraint vertical L93
  constraint horizontal L94
  constraint vertical L95
  constraint horizontal L96
  constraint vertical L97
  constraint coincident L85 L98.end
  constraint horizontal L186
  constraint vertical L99
  constraint horizontal L171
  constraint vertical L100
  constraint perpendicular L7 L101
  constraint horizontal L102
  constraint vertical L190
  constraint horizontal L103
  constraint vertical L173
  constraint horizontal L108
  constraint vertical L109
  constraint horizontal L110
  constraint coincident L110.start L173
  constraint coincident L104 L110.start
  constraint horizontal L111
  constraint vertical L112
  constraint vertical L113
  constraint coincident L107 L112.end
  constraint horizontal L114
  constraint vertical L115
  constraint vertical L116
  constraint coincident L107 L116.end
  constraint horizontal L117
  constraint horizontal L118
  constraint vertical L119
  constraint coincident L117.start L190
  constraint coincident L106 L117.start
  constraint horizontal L120
  constraint vertical L121
  constraint horizontal L122
  constraint coincident L106 L122.start
  constraint vertical L123
  constraint horizontal L124
  constraint vertical L125
  constraint coincident L105 L125.end
  constraint vertical L126
  constraint horizontal L127
  constraint vertical L128
  constraint coincident L105 L128.end
  constraint horizontal L129
  constraint vertical L130
  constraint horizontal L131
  constraint coincident L104 L129.start
  constraint horizontal L136
  constraint vertical L137
  constraint horizontal L138
  constraint coincident L75 L137.end
  constraint coincident L104 L137.end
  constraint horizontal L139
  constraint horizontal L140
  constraint vertical L141
  constraint coincident L73 L139.start
  constraint coincident L132 L139.start
  constraint vertical L142
  constraint horizontal L143
  constraint vertical L144
  constraint coincident L107 L142.end
  constraint coincident L79 L142.end
  constraint vertical L145
  constraint horizontal L146
  constraint vertical L147
  constraint coincident L107 L145.end
  constraint coincident L77 L145.end
  constraint horizontal L148
  constraint vertical L149
  constraint horizontal L150
  constraint coincident L73 L149.end
  constraint coincident L106 L149.end
  constraint horizontal L151
  constraint horizontal L152
  constraint vertical L153
  constraint coincident L75 L151.start
  constraint coincident L134 L151.start
  constraint vertical L154
  constraint horizontal L155
  constraint vertical L156
  constraint coincident L135 L154.end
  constraint coincident L77 L154.end
  constraint vertical L157
  constraint horizontal L158
  constraint vertical L159
  constraint coincident L135 L157.end
  constraint coincident L79 L157.end
  constraint coincident L77 L10.start
  constraint collinear L162 L173
  constraint collinear L163 L186
  constraint coincident L75 L164.end
  constraint coincident L75 L166.end
  constraint coincident L8.start L186
  constraint coincident L77 L9.end
  constraint collinear L171 L176
  constraint collinear L173 L174
  constraint collinear L176 L177
  constraint coincident L40 L179.start
  constraint collinear L178 L179
  constraint coincident L132 L179.end
  constraint coincident L68 L180.start
  constraint collinear L179 L180
  constraint coincident L135 L183.end
  constraint coincident L69 L181.start
  constraint collinear L181 L182
  constraint coincident L41 L183.start
  constraint collinear L182 L183
  constraint collinear L186 L187
  constraint collinear L190 L191
  measures "d1" distance of L0.start L0.end
  measures "d2" distance of L0.start L2.end
  measures "d3" diameter of A0
  measures "d4" distance of L4.start L4.end
  measures "d5" distance of L5.start L5.end
  measures "d6" distance of L6.start L6.end
  measures "d7" distance of L7.start L7.end
  measures "d8" distance of L13.start L13.end
  measures "d9" distance of L13.start L14.end
  measures "d10" distance of L15.start L15.end
  measures "d11" distance of L15.end L16.end
  measures "d12" distance of L17.start L17.end
  measures "d13" distance of L17.end L18.end
  measures "d14" distance of L19.start L19.end
  measures "d15" distance of L19.end L20.end
  measures "d18" angle of L25 L26
  measures "d20" angle of L31 L32
  measures "d24" distance of L1.end L39.end
  measures "d25" distance of L1.end L41.end
  measures "d26" distance of L2.end L45.end
  measures "d27" distance of L2.end L43.end
  measures "d28" distance of L0.start L47.end
  measures "d29" distance of L0.start L49.end
  measures "d30" distance of L0.end L53.end
  measures "d31" distance of L0.end L51.end
  measures "d32" distance of L2.end L57.end
  measures "d33" distance of L2.end L55.end
  measures "d34" distance of L0.start L59.end
  measures "d35" distance of L0.start L61.end
  measures "d36" distance of L0.end L63.end
  measures "d37" distance of L0.end L65.end
  measures "d38" distance of L1.end L67.end
  measures "d39" distance of L1.end L69.end
  measures "d40" distance of L4.start L71.end
  measures "d41" distance of L71.end L72.end
  measures "d42" distance of L5.start L76.end
  measures "d43" distance of L76.end L77.end
  measures "d44" distance of L76.end L79.end
  measures "d47" distance of L5.start L84.end
  measures "d48" distance of L84.end L86.start
  measures "d49" distance of L6.start L98.end
  measures "d50" distance of L98.end L100.start
  measures "d51" distance of L98.end L99.start
  measures "d52" distance of L7.start L101.end
  measures "d53" distance of L101.end L102.end
  measures "d54" distance of L101.end L103.end
extrude "Extrude1" add sketch "Sketch1" along normal blind 110
equation "length = 110 mm"
equation "d56 = length"

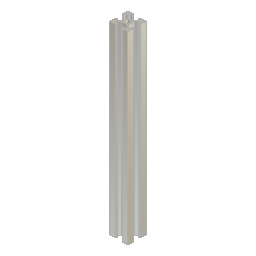
design "towerExtrusionsFront"
Autodesk Fusion 360 part; units mm, degrees